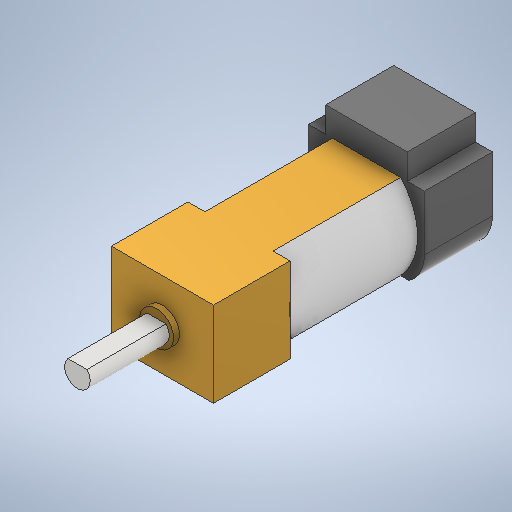
# Autodesk Inventor part: MercuryN20
Saved by Autodesk Inventor 2025 (Build 290162000, 162)
## iProperties
Created: 2025-05-20
Part Number: MercuryN20
Material: 一般
Document SubType Name: Modeling
Designer: daisuke
Density: 1 g/cm^3
Appearance: 既定
Author: daisuke
Autodesk Inventor part; units mm, degrees
ref_plane "YZ Plane" through (0, 0, 0) normal (1, 0, 0) x (0, 1, 0)
ref_plane "XZ Plane" through (0, 0, 0) normal (0, 1, 0) x (-1, 0, 0)
ref_plane "XY Plane" through (0, 0, 0) normal (0, 0, 1) x (1, 0, 0)
sketch "スケッチ1" plane through (0, 0, 0) normal (0, 0, 1) x (1, 0, 0)
  line L0 (-6, 5) -> (6, 5)
  line L1 (6, 5) -> (6, -5)
  line L2 (6, -5) -> (-6, -5)
  line L3 (-6, -5) -> (-6, 5)
  point P0 (0, 0)
  point P1 (0, -5)
  point P2 (6, 0)
  dimension "d0" = 12
  dimension "d1" = 10
  constraints: 8 end point, 2 midpoint, 2 parallel, 1 horizontal, 1 horizontal alignment, 1 perpendicular, 1 vertical alignment
  measures "d0" distance of L1.end L2.end
  measures "d1" distance of L0.end L1.end
extrude "ギヤボックス" add sketch "スケッチ1" against normal blind 9
sketch "スケッチ2" plane through (0, 0, 0) normal (0, 0, 1) x (1, 0, 0)
  circle A0 centre (0, 0) radius 1.5
  line L0 (-1.118, 1) -> (1.118, 1)
  circle A1 centre (0, 0) radius 2
  dimension "d4" = 3
  dimension "d5" = 1
  dimension "d6" = 4
  constraints: 2 centre point, 2 coincident, 2 end point, 2 point on circle, 1 horizontal
  measures "d4" diameter of A0
  measures "d5" distance from line of point (0, 0) L0
  measures "d6" diameter of A1
extrude "軸受け" add sketch "スケッチ2" along normal blind 0.7 contours A0 L0 | L0 A0 | A1
extrude "軸" add sketch "スケッチ2" along normal blind 10 contours A0 L0 picked at (0.0594, 0.1702)
sketch "スケッチ3" plane through (0, 0, -9) normal (0, 0, -1) x (-1, 0, 0)
  line L0 (6, 5) -> (-6, 5) projected
  line L1 (-6, -5) -> (6, -5) projected
  line L2 (-4, 5) -> (4, 5)
  line L3 (4, 5) -> (4, -5)
  line L4 (4, -5) -> (-4, -5)
  line L5 (-4, -5) -> (-4, 5)
  arc A0 (-4, 5) -> (-4, -5) centre (1.25, 0) ccw
  arc A1 (4, -5) -> (4, 5) centre (-1.25, 0) ccw
  line L6 (-6, 5) -> (-6, -5) projected
  line L7 (6, -5) -> (6, 5) projected
  line L8 (0, 7.0621) -> (0, -7.0621) construction
  line L9 (-6, 7.0625) -> (-6, -7.0625) construction
  line L10 (6, -7.0752) -> (6, 7.0489) construction
  point P0 (0, 0)
  point P1 (0, 5)
  point P2 (0, 0)
  point P3 (4, 5)
  point P4 (-4, -5)
  dimension "d11" = 8
  dimension "d15" = 12
  constraints: 14 end point, 4 point on circle, 2 centre point, 2 midpoint, 2 parallel, 2 point on line, 2 tangent, 2 vertical, 1 coincident, 1 horizontal, 1 perpendicular, 1 vertical alignment, 1 other
  measures "d11" distance between parallel lines of L3 L5
  measures "d15" distance from line of L10.start L9
extrude "モーター" add sketch "スケッチ3" along normal blind 15 contours L3 L1 L5 L0 | A1 L3 | L5 A0
sketch "スケッチ4" plane through (0, 0, -24) normal (0, 0, -1) x (-1, 0, 0)
  line L0 (-6.8, -5) -> (6.8, -5)
  line L1 (6.8, -5) -> (6.8, 5)
  line L2 (6.8, 5) -> (-6.8, 5)
  line L3 (-6.8, 5) -> (-6.8, -5)
  arc A0 (-6.8, -1.5) -> (-4.998, -5) centre (-2.5, -1.5) ccw
  arc A1 (4.998, -5) -> (6.8, -1.5) centre (2.5, -1.5) ccw
  line L4 (-4, -5) -> (4, -5) projected
  line L5 (0, 7.2835) -> (0, -7.2835) construction
  line L6 (-4.8, 5) -> (4.8, 5)
  line L7 (4.8, 5) -> (4.8, 8)
  line L8 (4.8, 8) -> (-4.8, 8)
  line L9 (-4.8, 8) -> (-4.8, 5)
  line L10 (4, 5) -> (-4, 5) projected
  point P0 (0, 0)
  point P1 (0, -5)
  point P2 (0, 0)
  point P3 (0, 8)
  dimension "d16" = 13.6
  dimension "d17" = 9.6
  dimension "d18" = 13
  dimension "d19" = 3.5
  dimension "d20" = 2.5
  constraints: 18 end point, 5 point on line, 4 parallel, 4 point on circle, 3 midpoint, 2 centre point, 2 collinear, 2 horizontal, 2 horizontal alignment, 2 perpendicular, 2 vertical alignment, 1 coincident, 1 symmetric about line, 1 tangent, 1 vertical
  measures "d16" distance between parallel lines of L1 L3
  measures "d17" distance of L7.end L8.end
  measures "d18" distance between parallel lines of L0 L8
  measures "d19" distance from line of L0 A0.centre
  measures "d20" distance from line of L5 A0.centre
extrude "エンコーダ" add sketch "スケッチ4" along normal blind 8 contours A0 L3 L2 L1 A1 L0 | L9 L8 L7 L2
